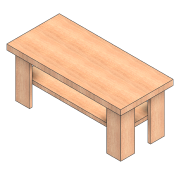
# Autodesk Inventor part: Sto u dnevnoj sobi
Saved by Autodesk Inventor 2020.2 (Build 242310000, 310)
## iProperties
Created: 2020-10-09
Part Number: Sto u dnevnoj sobi
Material: Wood (Birch)
Document SubType Name: Modeling
Designer: User
Density: 0.55 g/cm^3
Appearance: Birch - Natural Polished
Author: User
Autodesk Inventor part; units mm, degrees
ref_plane "YZ Plane" through (0, 0, 0) normal (1, 0, 0) x (0, 1, 0)
sketch "Sketch1" plane through (0, 0, 0) normal (0, 1, 0) x (-1, 0, 0)
  line L0 (-650, -300) -> (650, -300)
  line L1 (650, -300) -> (650, 300)
  line L2 (650, 300) -> (-650, 300)
  line L3 (-650, 300) -> (-650, -300)
  line L4 (-650, -300) -> (650, 300) construction
  line L5 (650, -300) -> (-650, 300) construction
  line L6 (650, 300) -> (600, 300)
  line L7 (600, 250) -> (570, 250)
  line L8 (570, 220) -> (570, 90)
  line L9 (570, 90) -> (600, 90)
  line L10 (600, 90) -> (600, 250)
  line L11 (600, 250) -> (440, 250)
  line L12 (440, 250) -> (440, 220)
  line L13 (440, 220) -> (570, 220)
  line L14 (600, 220) -> (600, 250)
  line L15 (650, -300) -> (600, -300)
  line L16 (650, -250) -> (650, -300)
  line L17 (600, -250) -> (440, -250)
  line L18 (440, -250) -> (440, -220)
  line L19 (440, -220) -> (570, -220)
  line L20 (600, -220) -> (600, -250)
  line L21 (600, -250) -> (570, -250)
  line L22 (570, -220) -> (570, -90)
  line L23 (570, -90) -> (600, -90)
  line L24 (600, -90) -> (600, -250)
  line L25 (-650, 300) -> (-600, 300)
  line L26 (-650, 250) -> (-650, 300)
  line L27 (-600, 250) -> (-570, 250)
  line L28 (-570, 220) -> (-570, 90)
  line L29 (-570, 90) -> (-600, 90)
  line L30 (-600, 90) -> (-600, 250)
  line L31 (-600, 250) -> (-440, 250)
  line L32 (-440, 250) -> (-440, 220)
  line L33 (-440, 220) -> (-570, 220)
  line L34 (-600, 220) -> (-600, 250)
  line L35 (-650, -300) -> (-600, -300)
  line L36 (-650, -250) -> (-650, -300)
  line L37 (-600, -250) -> (-440, -250)
  line L38 (-440, -250) -> (-440, -220)
  line L39 (-440, -220) -> (-570, -220)
  line L40 (-600, -220) -> (-600, -250)
  line L41 (-600, -250) -> (-570, -250)
  line L42 (-570, -220) -> (-570, -90)
  line L43 (-570, -90) -> (-600, -90)
  line L44 (-600, -90) -> (-600, -250)
  point P0 (0, 0)
  dimension "d0" = 1300
  dimension "d1" = 600
  dimension "d4" = 30
  dimension "d5" = 160
  dimension "d6" = 30
  dimension "d7" = 50
  dimension "d8" = 50
  dimension "d9" = 50
  dimension "d10" = 50
  dimension "d11" = 30
  dimension "d12" = 160
  dimension "d13" = 160
  dimension "d14" = 30
  constraints: 90 end point, 18 parallel, 12 horizontal, 9 perpendicular, 2 midpoint, 1 point on line
  measures "d0" distance of L2.end L1.end
  measures "d1" distance of L1.end L0.end
  measures "d4" distance of L9.end L8.end
  measures "d5" distance of L14.start L12.end
  measures "d6" distance of L12.end L11.end
  measures "d7" distance of L17.start L16.start
  measures "d8" distance of L15.end L17.start
  measures "d9" distance of L27.start L26.start
  measures "d10" distance of L25.end L27.start
  measures "d11" distance of L28.end L29.end
  measures "d12" distance of L27.end L28.end
  measures "d13" distance of L32.end L34.start
  measures "d14" distance of L31.end L32.end
extrude "Extrusion1" add sketch "Sketch1" along normal blind 60 contours L3 L2 L1 L0 | L10 L9 L8 L13 L12 L11 L7 | L17 L18 L19 L22 L23 L24 L20 | L27 L31 L32 L33 L28 L29 L30 | L40 L44 L43 L42 L39 L38 L37
ref_plane "Work Plane1" through (0, 0, 0) normal (0, -1, 0) x (1, 0, 0)
sketch "Sketch2" plane through (0, 0, 0) normal (0, -1, 0) x (1, 0, 0)
  line L0 (650, 300) -> (650, -300) projected
  line L1 (650, 300) -> (600, 300)
  line L2 (650, 250) -> (650, 300)
  line L3 (650, -300) -> (600, -300)
  line L4 (650, -250) -> (650, -300)
  line L5 (-650, -300) -> (-650, 300) projected
  line L6 (-650, -300) -> (-600, -300)
  line L7 (-650, -250) -> (-650, -300)
  line L8 (-650, 300) -> (-600, 300)
  line L9 (-650, 250) -> (-650, 300)
  line L10 (-600, -250) -> (-440, -250)
  line L11 (-440, -250) -> (-440, -220)
  line L12 (-440, -220) -> (-570, -220)
  line L13 (-600, -220) -> (-600, -250)
  line L14 (-600, -250) -> (-570, -250)
  line L15 (-570, -220) -> (-570, -90)
  line L16 (-570, -90) -> (-600, -90)
  line L17 (-600, -90) -> (-600, -250)
  line L18 (-600, 250) -> (-440, 250)
  line L19 (-440, 250) -> (-440, 220)
  line L20 (-440, 220) -> (-570, 220)
  line L21 (-600, 220) -> (-600, 250)
  line L22 (-600, 250) -> (-570, 250)
  line L23 (-570, 220) -> (-570, 90)
  line L24 (-570, 90) -> (-600, 90)
  line L25 (-600, 90) -> (-600, 250)
  line L26 (600, -250) -> (440, -250)
  line L27 (440, -250) -> (440, -220)
  line L28 (440, -220) -> (570, -220)
  line L29 (600, -220) -> (600, -250)
  line L30 (600, -250) -> (570, -250)
  line L31 (570, -220) -> (570, -90)
  line L32 (570, -90) -> (600, -90)
  line L33 (600, -90) -> (600, -250)
  line L34 (600, 250) -> (570, 250)
  line L35 (570, 220) -> (570, 90)
  line L36 (570, 90) -> (600, 90)
  line L37 (600, 90) -> (600, 250)
  line L38 (600, 250) -> (440, 250)
  line L39 (440, 250) -> (440, 220)
  line L40 (440, 220) -> (570, 220)
  line L41 (600, 220) -> (600, 250)
  point P0 (0, 0)
  dimension "d18" = 50
  dimension "d19" = 50
  dimension "d20" = 50
  dimension "d21" = 50
  dimension "d22" = 50
  dimension "d23" = 50
  dimension "d24" = 50
  dimension "d25" = 50
  dimension "d26" = 160
  dimension "d27" = 30
  dimension "d28" = 30
  dimension "d29" = 160
  dimension "d30" = 160
  dimension "d31" = 30
  dimension "d32" = 30
  dimension "d33" = 160
  dimension "d34" = 160
  dimension "d35" = 30
  dimension "d36" = 30
  dimension "d37" = 160
  constraints: 80 end point, 16 parallel, 12 horizontal, 8 perpendicular, 3 point on line
  measures "d18" distance of L2.start L34.start
  measures "d19" distance of L34.start L1.end
  measures "d20" distance of L26.start L4.start
  measures "d21" distance of L3.end L26.start
  measures "d22" distance of L7.start L10.start
  measures "d23" distance of L10.start L6.end
  measures "d24" distance of L18.start L9.start
  measures "d25" distance of L8.end L18.start
  measures "d26" distance of L13.start L11.end
  measures "d27" distance of L11.end L10.end
  measures "d28" distance of L16.end L15.end
  measures "d29" distance of L15.end L14.end
  measures "d30" distance of L19.end L21.start
  measures "d31" distance of L18.end L19.end
  measures "d32" distance of L23.end L24.end
  measures "d33" distance of L22.end L23.end
  measures "d34" distance of L27.end L29.start
  measures "d35" distance of L26.end L27.end
  measures "d36" distance of L31.end L32.end
  measures "d37" distance of L30.end L31.end
extrude "Extrusion2" add sketch "Sketch2" along normal blind 500
ref_plane "Work Plane2" through (0, -250, 0) normal (0, -1, 0) x (1, 0, 0)
sketch "Sketch3" plane through (0, -250, 0) normal (0, -1, 0) x (1, 0, 0)
  line L0 (570, 220) -> (-570, 220)
  line L1 (-570, 220) -> (-570, -220)
  line L2 (-570, -220) -> (570, -220)
  line L3 (570, -220) -> (570, 220)
  point P0 (0, 0)
  constraints: 8 end point, 2 parallel, 1 horizontal, 1 perpendicular
extrude "Extrusion3" add sketch "Sketch3" along normal blind 20 and the other way blind 20
body "Solid1"
